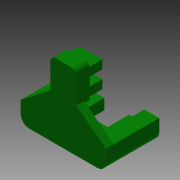
# Autodesk Inventor part: PiCam Holder
Saved by Autodesk Inventor 2014 (Build 180170000, 170)
## iProperties
Created: 2016-02-04
Part Number: PiCam Holder
Material: Generic
Document SubType Name: Modeling
Designer: Paul
Density: 1 g/cm^3
Appearance: Dark Green
Author: Paul
Autodesk Inventor part; units mm, degrees
ref_plane "YZ Plane" through (0, 0, 0) normal (1, 0, 0) x (0, 1, 0)
ref_plane "XZ Plane" through (0, 0, 0) normal (0, 1, 0) x (-1, 0, 0)
ref_plane "XY Plane" through (0, 0, 0) normal (0, 0, 1) x (1, 0, 0)
sketch "Sketch2" plane through (0, 0, 0) normal (0, 1, 0) x (-1, 0, 0)
  line L0 (16, -6.6684) -> (16, 6.6684)
  line L1 (9.675, -1.4184) -> (12.925, -1.4184)
  line L2 (12.925, -1.4184) -> (12.925, -2.9684)
  line L3 (12.925, -2.9684) -> (4.35, -2.9684)
  line L4 (4.35, -2.9684) -> (4.35, -4.6684)
  line L5 (4.35, -4.6684) -> (-4.35, -4.6684)
  line L6 (-4.35, -4.6684) -> (-4.35, -3.6684)
  line L7 (-9.675, -2.9684) -> (-12.925, -2.9684)
  line L8 (-12.925, -2.9684) -> (-12.925, -1.4184)
  line L9 (-12.925, -1.4184) -> (-9.675, -1.4184)
  line L10 (-9.675, -1.4184) -> (-9.675, 0.5816)
  line L11 (-9.675, 0.5816) -> (-14.925, 0.5816)
  line L12 (-14.925, 0.5816) -> (-14.925, -6.6684)
  line L13 (14.925, -6.6684) -> (14.925, 0.5816)
  line L14 (14.925, 0.5816) -> (9.675, 0.5816)
  line L15 (9.675, 0.5816) -> (9.675, -1.4184)
  line L16 (-9.675, -2.9684) -> (-9.675, -3.6684)
  line L17 (-9.675, -3.6684) -> (-4.35, -3.6684)
  line L18 (-16, -6.6684) -> (16, -6.6684)
  line L19 (0, 0) -> (0, -6.6684) construction
  dimension "d2" = 25.25
  dimension "d5" = 0.95
  dimension "d11" = 0.7
  dimension "d13" = 2
  dimension "d14" = 2
  dimension "d16" = 1.1
  dimension "d22" = 8.1
  dimension "d23" = 3.25
  dimension "d24" = 2
  constraints: 40 end point, 12 parallel, 6 equal length, 5 perpendicular, 2 point on line, 1 midpoint, 2 other
  measures "d11" distance between parallel lines of L17 L7
  measures "d13" distance between parallel lines of L12 L8
  measures "d14" distance of L9.end L10.end
  measures "d23" distance of L1.start L1.end
  measures "d24" distance between parallel lines of L18 L5
extrude "Extrusion2" add sketch "Sketch2" along normal blind 16
sketch "Sketch4" plane through (0, 16, 0) normal (0, 1, 0) x (1, 0, 0)
  line L0 (-4.35, 4.6684) -> (4.35, 4.6684) projected
  line L1 (14.925, 6.6684) -> (-14.925, 6.6684) projected
  line L2 (-4.35, 4.6684) -> (-4.35, 6.6684)
  line L3 (4.35, 4.6684) -> (4.35, 6.6684)
  point P0 (0, 0)
  constraints: 4 end point, 2 perpendicular, 2 point on line
extrude "Extrusion4" cut sketch "Sketch4" against normal blind 6.5
sketch "Sketch5" plane through (0, 0, 0) normal (0, -1, 0) x (1, 0, 0)
  line L0 (-9.675, -1.4184) -> (-12.925, -1.4184) projected
  line L1 (-9.675, 0.5816) -> (-9.675, -1.4184) projected
  line L2 (-14.925, 0.5816) -> (-9.675, 0.5816) projected
  line L3 (-14.925, -6.6684) -> (-14.925, 0.5816) projected
  line L4 (14.925, -6.6684) -> (-14.925, -6.6684) projected
  line L5 (14.925, 0.5816) -> (14.925, -6.6684) projected
  line L6 (9.675, 0.5816) -> (14.925, 0.5816) projected
  line L7 (9.675, -1.4184) -> (9.675, 0.5816) projected
  line L8 (12.925, -1.4184) -> (9.675, -1.4184) projected
  line L9 (12.925, -2.9684) -> (12.925, -1.4184) projected
  line L10 (9.675, -2.9684) -> (12.925, -2.9684) projected
  line L11 (9.675, -3.6684) -> (9.675, -2.9684) projected
  line L12 (4.35, -3.6684) -> (9.675, -3.6684) projected
  line L13 (4.35, -4.6684) -> (4.35, -3.6684) projected
  line L14 (-4.35, -4.6684) -> (4.35, -4.6684) projected
  line L15 (-4.35, -2.9684) -> (-4.35, -4.6684) projected
  line L16 (-12.925, -2.9684) -> (-4.35, -2.9684) projected
  line L17 (-12.925, -1.4184) -> (-12.925, -2.9684) projected
  line L18 (-14.925, 0.5816) -> (-4.55, 8.5816)
  line L19 (-4.55, 8.5816) -> (-4.55, 19.3316)
  line L20 (-4.55, 19.3316) -> (4.55, 19.3316)
  line L21 (4.55, 19.3316) -> (4.55, 8.5816)
  line L22 (4.55, 8.5816) -> (14.925, 0.5816)
  line L23 (0, -6.6684) -> (0, 19.3316) construction
  point P0 (0, 0)
  dimension "d27" = 9.5
  dimension "d28" = 26
  dimension "d29" = 8
  constraints: 12 end point, 3 parallel, 2 midpoint, 2 perpendicular, 1 point on line, 1 other
  measures "d28" distance between parallel lines of L4 L20
  measures "d29" distance from line of L18.end L2
extrude "Extrusion5" add sketch "Sketch5" along normal blind 2.75
sketch "Sketch6" plane through (0, 0, 0) normal (0, 1, 0) x (1, 0, 0)
  line L0 (-4.55, -19.3316) -> (-4.55, -8.5816) projected
  line L1 (4.55, -19.3316) -> (-4.55, -19.3316) projected
  line L2 (4.55, -8.5816) -> (4.55, -19.3316) projected
  line L3 (-4.55, -8.5816) -> (-4.55, -6.5316)
  line L4 (-4.55, -6.5316) -> (4.55, -6.5316)
  line L5 (4.55, -6.5316) -> (4.55, -8.5816)
  point P0 (0, 0)
  dimension "d32" = 13.2
  constraints: 6 end point, 2 parallel, 1 perpendicular
extrude "Extrusion6" add sketch "Sketch6" along normal blind 2
fillet "Fillet1" radius 2 4 edges at (-4.55, 1, 6.5316) (4.55, 1, 6.5316) (-4.55, -0.375, 19.3316) (4.55, -0.375, 19.3316)
sketch "Sketch7" plane through (0, 2, 0) normal (0, 1, 0) x (1, 0, 0)
  line L0 (4.55, -17.3316) -> (4.55, -8.5316) projected
  line L1 (2.55, -6.5316) -> (-2.55, -6.5316) projected
  line L2 (-4.55, -8.5316) -> (-4.55, -17.3316) projected
  line L3 (-2.55, -19.3316) -> (2.55, -19.3316) projected
  line L4 (-4, -11.4316) -> (4, -11.4316)
  line L5 (4, -8.4316) -> (-4, -8.4316)
  line L6 (-4, -14.4316) -> (4, -14.4316)
  line L7 (4, -17.4316) -> (-4, -17.4316)
  line L8 (-4.55, -12.9316) -> (4.55, -12.9316) construction
  line L9 (0, -6.5316) -> (0, -19.3316) construction
  line L10 (-4, -8.4316) -> (-4, -11.4316)
  line L11 (-4, -14.4316) -> (-4, -17.4316)
  line L12 (4, -8.4316) -> (4, -11.4316)
  line L13 (4, -14.4316) -> (4, -17.4316)
  point P0 (0, 0)
  dimension "d36" = 3
  dimension "d37" = 3
  dimension "d38" = 3
  dimension "d39" = 8
  constraints: 20 end point, 8 perpendicular, 4 midpoint, 1 parallel, 3 other
  measures "d36" distance between parallel lines of L6 L7
  measures "d37" distance between parallel lines of L5 L4
  measures "d38" distance between parallel lines of L6 L4
  measures "d39" distance of L5.start L5.end
extrude "Extrusion7" add sketch "Sketch7" along normal blind 5
fillet "Fillet2" radius 3 2 edges at (14.925, 6.625, -6.6684) (-14.925, 6.625, -6.6684)
equation "\"d13\" = d14"
body "Solid1"
